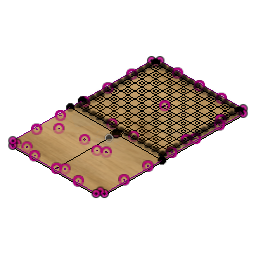
Bottom Plate (Autodesk Fusion 360 design; units mm, degrees)
Autodesk Fusion 360 part; units mm, degrees
note: some values were not read from the file. Set by a fixed rule: which sketch regions a step uses.
sketch "Sketch1" plane through (0, 0, 0) normal (0, 1, 0) x (1, 0, 0)
  line L0 (0, 0) -> (330, 0)
  line L1 (330, 0) -> (330, -530)
  line L2 (330, -530) -> (0, -530)
  line L3 (0, -530) -> (0, 0)
  dimension "d1" = 530
  dimension "d2" = 330
  measures "d1" distance of L0.start
extrude "Extrude1" add sketch "Sketch1" along normal blind 6
sketch "Sketch3" plane through (0, 6, 0) normal (0, 1, 0) x (-1, 0, 0)
  circle A0 centre (-7.5, 7.5) radius 1.5
  line L0 (0, 0) -> (0, 530)
  line L1 (-330, 0) -> (0, 0)
  circle A1 centre (-322.5, 7.5) radius 1.5
  circle A2 centre (-7.5, 93.3333) radius 1.5
  circle A3 centre (-322.5, 93.3333) radius 1.5
  circle A4 centre (-7.5, 179.1667) radius 1.5
  circle A5 centre (-322.5, 179.1667) radius 1.5
  circle A6 centre (-7.5, 265) radius 1.5
  circle A7 centre (-322.5, 265) radius 1.5
  circle A8 centre (-7.5, 350.8333) radius 1.5
  circle A9 centre (-322.5, 350.8333) radius 1.5
  circle A10 centre (-7.5, 436.6667) radius 1.5
  circle A11 centre (-322.5, 436.6667) radius 1.5
  circle A12 centre (-7.5, 522.5) radius 1.5
  circle A13 centre (-322.5, 522.5) radius 1.5
  circle A14 centre (-243.75, 7.5) radius 1.5
  circle A15 centre (-165, 7.5) radius 1.5
  circle A16 centre (-86.25, 7.5) radius 1.5
  circle A17 centre (-7.5, 7.5) radius 1.5
  circle A18 centre (-322.5, 522.5) radius 1.5
  circle A19 centre (-243.75, 522.5) radius 1.5
  circle A20 centre (-165, 522.5) radius 1.5
  circle A21 centre (-86.25, 522.5) radius 1.5
  circle A22 centre (-7.5, 522.5) radius 1.5
  dimension "d87" = 3
  dimension "d88" = 7.5
  dimension "d89" = 7.5
  dimension "d92" = -315
  dimension "d93" = 515
  dimension "d96" = 315
  dimension "d97" = 515
  measures "d87" diameter of A0
  measures "d88" distance of L0
extrude "Extrude3" cut sketch "Sketch3" against normal through all
sketch "Sketch4" plane through (0, 6, 0) normal (0, 1, 0) x (-1, 0, 0)
  line L0 (0, 530) -> (-330, 530)
  line L1 (-330, 530) -> (-330, 0)
  line L2 (-330, 0) -> (0, 0)
  line L3 (0, 0) -> (0, 530)
  line L4 (0, 530) -> (-15, 530)
  line L5 (-15, 530) -> (-15, 515)
  line L6 (-15, 515) -> (0, 515)
  line L7 (0, 515) -> (0, 530)
  line L8 (-330, 530) -> (-315, 530)
  line L9 (-315, 530) -> (-315, 515)
  line L10 (-315, 515) -> (-330, 515)
  line L11 (-330, 515) -> (-330, 530)
  line L12 (-330, 0) -> (-315, 0)
  line L13 (-315, 0) -> (-315, 15)
  line L14 (-315, 15) -> (-330, 15)
  line L15 (-330, 15) -> (-330, 0)
  line L16 (0, 0) -> (-15, 0)
  line L17 (-15, 0) -> (-15, 15)
  line L18 (-15, 15) -> (0, 15)
  line L19 (0, 15) -> (0, 0)
  circle A0 centre (-7.5, 265) radius 1.5
  circle A1 centre (-86.25, 7.5) radius 1.5
  circle A2 centre (-322.5, 93.3333) radius 1.5
  circle A3 centre (-322.5, 436.6667) radius 1.5
  circle A4 centre (-86.25, 522.5) radius 1.5
  circle A5 centre (-165, 522.5) radius 1.5
  circle A6 centre (-322.5, 350.8333) radius 1.5
  circle A7 centre (-322.5, 7.5) radius 1.5
  circle A8 centre (-7.5, 7.5) radius 1.5
  circle A9 centre (-7.5, 350.8333) radius 1.5
  circle A10 centre (-7.5, 179.1667) radius 1.5
  circle A11 centre (-165, 7.5) radius 1.5
  circle A12 centre (-322.5, 179.1667) radius 1.5
  circle A13 centre (-322.5, 522.5) radius 1.5
  circle A14 centre (-7.5, 522.5) radius 1.5
  circle A15 centre (-243.75, 522.5) radius 1.5
  circle A16 centre (-322.5, 265) radius 1.5
  circle A17 centre (-243.75, 7.5) radius 1.5
  circle A18 centre (-7.5, 93.3333) radius 1.5
  circle A19 centre (-7.5, 436.6667) radius 1.5
  dimension "d38" = 15
  dimension "d39" = 15
  dimension "d40" = 15
  dimension "d41" = 15
  dimension "d42" = 15
  dimension "d43" = 15
  dimension "d44" = 15
  dimension "d45" = 15
  measures "d44" distance of L2.end
  measures "d45" distance of L2.end
extrude "Extrude4" cut sketch "Sketch4" against normal blind 25 contours L0 L3 L4 L5 L6 L7 | L0 L1 L8 L9 L10 L11 | L2 L3 L16 L17 L18 L19 | L1 L2 L12 L13 L14 L15
sketch "Sketch5" plane through (0, 6, 0) normal (0, 1, 0) x (-1, 0, 0)
  line L0 (-315, 530) -> (-315, 515)
  line L1 (-315, 515) -> (-330, 515)
  line L2 (-330, 515) -> (-330, 15)
  line L3 (-330, 15) -> (-315, 15)
  line L4 (-315, 15) -> (-315, 0)
  line L5 (-315, 0) -> (-15, 0)
  line L6 (-15, 0) -> (-15, 15)
  line L7 (-15, 15) -> (0, 15)
  line L8 (0, 15) -> (0, 515)
  line L9 (0, 515) -> (-15, 515)
  line L10 (-15, 515) -> (-15, 530)
  line L11 (-15, 530) -> (-315, 530)
  line L12 (-126, 382) -> (-204, 382)
  line L13 (-204, 382) -> (-204, 284)
  line L14 (-204, 284) -> (-126, 284)
  line L15 (-126, 284) -> (-126, 382)
  circle A0 centre (-126, 382) radius 2.5
  circle A1 centre (-126, 284) radius 2.5
  circle A2 centre (-204, 284) radius 2.5
  circle A3 centre (-204, 382) radius 2.5
  line L16 (-165, 530) -> (-165, 382) construction
  circle A4 centre (-7.5, 436.6667) radius 1.5
  circle A5 centre (-7.5, 93.3333) radius 1.5
  circle A6 centre (-243.75, 7.5) radius 1.5
  circle A7 centre (-322.5, 265) radius 1.5
  circle A8 centre (-243.75, 522.5) radius 1.5
  circle A9 centre (-322.5, 179.1667) radius 1.5
  circle A10 centre (-165, 7.5) radius 1.5
  circle A11 centre (-7.5, 179.1667) radius 1.5
  circle A12 centre (-7.5, 350.8333) radius 1.5
  circle A13 centre (-322.5, 350.8333) radius 1.5
  circle A14 centre (-165, 522.5) radius 1.5
  circle A15 centre (-86.25, 522.5) radius 1.5
  circle A16 centre (-322.5, 436.6667) radius 1.5
  circle A17 centre (-322.5, 93.3333) radius 1.5
  circle A18 centre (-86.25, 7.5) radius 1.5
  circle A19 centre (-7.5, 265) radius 1.5
  dimension "d48" = 78
  dimension "d49" = 98
  dimension "d50" = 5
  dimension "d51" = 5
  dimension "d52" = 5
  dimension "d53" = 5
  dimension "d54" = 148
  measures "d49" distance of origin
  measures "d50" diameter of A0
  measures "d51" diameter of A1
  measures "d52" diameter of A2
  measures "d53" diameter of A3
extrude "Extrude5" cut sketch "Sketch5" against normal through all contours L12 L13 A3 | L12 L13 A3 | L12 L15 A0 | L12 L15 A0 | L13 L14 A2 | L13 L14 A2 | L14 L15 A1 | L14 L15 A1
sketch "Sketch6" plane through (0, 6, 0) normal (0, 1, 0) x (-1, 0, 0)
  circle A0 centre (-204, 284) radius 2.5
  circle A1 centre (-204, 382) radius 2.5
  circle A2 centre (-126, 284) radius 2.5
  circle A3 centre (-126, 382) radius 2.5
  line L0 (-315, 530) -> (-315, 515)
  line L1 (-315, 515) -> (-330, 515)
  line L2 (-330, 515) -> (-330, 15)
  line L3 (-330, 15) -> (-315, 15)
  line L4 (-315, 15) -> (-315, 0)
  line L5 (-315, 0) -> (-15, 0)
  line L6 (-15, 0) -> (-15, 15)
  line L7 (-15, 15) -> (0, 15)
  line L8 (0, 15) -> (0, 515)
  line L9 (0, 515) -> (-15, 515)
  line L10 (-15, 515) -> (-15, 530)
  line L11 (-15, 530) -> (-315, 530)
  line L12 (-45, 509) -> (-182, 509) construction
  line L13 (-182, 509) -> (-182, 394) construction
  line L14 (-182, 394) -> (-45, 394) construction
  line L15 (-45, 394) -> (-45, 509) construction
  circle A4 centre (-182, 509) radius 2
  circle A5 centre (-45, 509) radius 2
  circle A6 centre (-45, 394) radius 2
  circle A7 centre (-182, 394) radius 2
  circle A8 centre (-7.5, 436.6667) radius 1.5
  circle A9 centre (-7.5, 93.3333) radius 1.5
  circle A10 centre (-243.75, 7.5) radius 1.5
  circle A11 centre (-322.5, 265) radius 1.5
  circle A12 centre (-243.75, 522.5) radius 1.5
  circle A13 centre (-322.5, 179.1667) radius 1.5
  circle A14 centre (-165, 7.5) radius 1.5
  circle A15 centre (-7.5, 179.1667) radius 1.5
  circle A16 centre (-7.5, 350.8333) radius 1.5
  circle A17 centre (-322.5, 350.8333) radius 1.5
  circle A18 centre (-165, 522.5) radius 1.5
  circle A19 centre (-86.25, 522.5) radius 1.5
  circle A20 centre (-322.5, 436.6667) radius 1.5
  circle A21 centre (-322.5, 93.3333) radius 1.5
  circle A22 centre (-86.25, 7.5) radius 1.5
  circle A23 centre (-7.5, 265) radius 1.5
  dimension "d56" = 115
  dimension "d57" = 137
  dimension "d58" = 4
  dimension "d59" = 21
  dimension "d60" = 45
  measures "d58" diameter of A4
  measures "d59" distance of L11 L12
  measures "d60" distance of L8 L15
extrude "Extrude6" cut sketch "Sketch6" against normal through all contours A4 | A5 | A6 | A7
sketch "Sketch9" plane through (0, 6, 0) normal (0, 1, 0) x (-1, 0, 0)
  circle A0 centre (-45, 394) radius 2
  circle A1 centre (-182, 394) radius 2
  circle A2 centre (-45, 509) radius 2
  circle A3 centre (-182, 509) radius 2
  circle A4 centre (-204, 284) radius 2.5
  circle A5 centre (-204, 382) radius 2.5
  circle A6 centre (-126, 284) radius 2.5
  circle A7 centre (-126, 382) radius 2.5
  circle A8 centre (-7.5, 436.6667) radius 1.5
  circle A9 centre (-7.5, 93.3333) radius 1.5
  circle A10 centre (-243.75, 7.5) radius 1.5
  circle A11 centre (-322.5, 265) radius 1.5
  circle A12 centre (-243.75, 522.5) radius 1.5
  circle A13 centre (-322.5, 179.1667) radius 1.5
  circle A14 centre (-165, 7.5) radius 1.5
  circle A15 centre (-7.5, 179.1667) radius 1.5
  circle A16 centre (-7.5, 350.8333) radius 1.5
  circle A17 centre (-322.5, 350.8333) radius 1.5
  circle A18 centre (-165, 522.5) radius 1.5
  circle A19 centre (-86.25, 522.5) radius 1.5
  circle A20 centre (-322.5, 436.6667) radius 1.5
  circle A21 centre (-322.5, 93.3333) radius 1.5
  circle A22 centre (-86.25, 7.5) radius 1.5
  circle A23 centre (-7.5, 265) radius 1.5
  line L0 (-315, 530) -> (-315, 515)
  line L1 (-315, 515) -> (-330, 515)
  line L2 (-330, 515) -> (-330, 15)
  line L3 (-330, 15) -> (-315, 15)
  line L4 (-315, 15) -> (-315, 0)
  line L5 (-315, 0) -> (-15, 0)
  line L6 (-15, 0) -> (-15, 15)
  line L7 (-15, 15) -> (0, 15)
  line L8 (0, 15) -> (0, 515)
  line L9 (0, 515) -> (-15, 515)
  line L10 (-15, 515) -> (-15, 530)
  line L11 (-15, 530) -> (-315, 530)
  circle A24 centre (-310, 75) radius 2
  circle A25 centre (-310, 200) radius 2
  circle A26 centre (-165, 132.643) radius 2.5
  line L12 (-126, 284) -> (-126, 382) construction
  line L13 (-204, 284) -> (-204, 382) construction
  line L14 (-204, 333) -> (-126, 333) construction
  line L15 (-165, 307.643) -> (-165, 132.643) construction
  line L16 (-165, 307.643) -> (-165, 333) construction
  circle A27 centre (-165, 307.643) radius 15 construction
  dimension "d98" = 4
  dimension "d99" = 4
  dimension "d100" = 20
  dimension "d101" = 20
  dimension "d102" = 75
  dimension "d103" = 200
  dimension "d104" = 5
  dimension "d105" = 175
  dimension "d108" = 23.643
  dimension "d109" = 30
  measures "d98" diameter of A24
  measures "d99" diameter of A25
  measures "d104" diameter of A26
  measures "d109" diameter of A27
extrude "Extrude7" cut sketch "Sketch9" against normal blind 10 contours A24 | A25 | A26
sketch "Sketch7" plane through (0, 6, 0) normal (0, 1, 0) x (-1, 0, 0)
  circle A0 centre (-45, 394) radius 2
  circle A1 centre (-182, 394) radius 2
  circle A2 centre (-45, 509) radius 2
  circle A3 centre (-182, 509) radius 2
  circle A4 centre (-204, 284) radius 2.5
  circle A5 centre (-204, 382) radius 2.5
  circle A6 centre (-126, 284) radius 2.5
  circle A7 centre (-126, 382) radius 2.5
  line L0 (-315, 530) -> (-315, 515)
  line L1 (-315, 515) -> (-330, 515)
  line L2 (-330, 515) -> (-330, 15)
  line L3 (-330, 15) -> (-315, 15)
  line L4 (-315, 15) -> (-315, 0)
  line L5 (-315, 0) -> (-15, 0)
  line L6 (-15, 0) -> (-15, 15)
  line L7 (-15, 15) -> (0, 15)
  line L8 (0, 15) -> (0, 515)
  line L9 (0, 515) -> (-15, 515)
  line L10 (-15, 515) -> (-15, 530)
  line L11 (-15, 530) -> (-315, 530)
  line L12 (-15, 15) -> (-315, 15)
  line L13 (-315, 15) -> (-315, 290)
  line L14 (-315, 290) -> (-15, 290)
  line L15 (-15, 290) -> (-15, 15)
  line L16 (-15, 40) -> (-315, 40)
  line L17 (-15, 65) -> (-315, 65)
  line L18 (-15, 90) -> (-315, 90)
  line L19 (-15, 115) -> (-315, 115)
  line L20 (-15, 140) -> (-315, 140)
  line L21 (-15, 165) -> (-315, 165)
  line L22 (-15, 190) -> (-315, 190)
  line L23 (-15, 215) -> (-315, 215)
  line L24 (-15, 240) -> (-315, 240)
  line L25 (-15, 265) -> (-315, 265)
  line L26 (-32.5, 32.5) -> (-22.5, 32.5)
  line L27 (-22.5, 32.5) -> (-22.5, 22.5)
  line L28 (-22.5, 22.5) -> (-32.5, 22.5)
  line L29 (-32.5, 22.5) -> (-32.5, 32.5)
  line L30 (-15, 290) -> (-315, 290)
  line L31 (-40, 290) -> (-40, 15)
  line L32 (-65, 290) -> (-65, 15)
  line L33 (-90, 290) -> (-90, 15)
  line L34 (-115, 290) -> (-115, 15)
  line L35 (-140, 290) -> (-140, 15)
  line L36 (-165, 290) -> (-165, 15)
  line L37 (-190, 290) -> (-190, 15)
  line L38 (-215, 290) -> (-215, 15)
  line L39 (-240, 290) -> (-240, 15)
  line L40 (-265, 290) -> (-265, 15)
  line L41 (-290, 290) -> (-290, 15)
  line L42 (-315, 290) -> (-315, 15)
  line L43 (-72.5, 22.5) -> (-82.5, 22.5)
  line L44 (-72.5, 32.5) -> (-72.5, 22.5)
  line L45 (-82.5, 32.5) -> (-72.5, 32.5)
  line L46 (-82.5, 22.5) -> (-82.5, 32.5)
  line L47 (-122.5, 22.5) -> (-132.5, 22.5)
  line L48 (-122.5, 32.5) -> (-122.5, 22.5)
  line L49 (-132.5, 32.5) -> (-122.5, 32.5)
  line L50 (-132.5, 22.5) -> (-132.5, 32.5)
  line L51 (-172.5, 22.5) -> (-182.5, 22.5)
  line L52 (-172.5, 32.5) -> (-172.5, 22.5)
  line L53 (-182.5, 32.5) -> (-172.5, 32.5)
  line L54 (-182.5, 22.5) -> (-182.5, 32.5)
  line L55 (-222.5, 22.5) -> (-232.5, 22.5)
  line L56 (-222.5, 32.5) -> (-222.5, 22.5)
  line L57 (-232.5, 32.5) -> (-222.5, 32.5)
  line L58 (-232.5, 22.5) -> (-232.5, 32.5)
  line L59 (-272.5, 22.5) -> (-282.5, 22.5)
  line L60 (-272.5, 32.5) -> (-272.5, 22.5)
  line L61 (-282.5, 32.5) -> (-272.5, 32.5)
  line L62 (-282.5, 22.5) -> (-282.5, 32.5)
  line L63 (-22.5, 72.5) -> (-32.5, 72.5)
  line L64 (-22.5, 82.5) -> (-22.5, 72.5)
  line L65 (-32.5, 82.5) -> (-22.5, 82.5)
  line L66 (-32.5, 72.5) -> (-32.5, 82.5)
  line L67 (-72.5, 72.5) -> (-82.5, 72.5)
  line L68 (-72.5, 82.5) -> (-72.5, 72.5)
  line L69 (-82.5, 82.5) -> (-72.5, 82.5)
  line L70 (-82.5, 72.5) -> (-82.5, 82.5)
  line L71 (-122.5, 72.5) -> (-132.5, 72.5)
  line L72 (-122.5, 82.5) -> (-122.5, 72.5)
  line L73 (-132.5, 82.5) -> (-122.5, 82.5)
  line L74 (-132.5, 72.5) -> (-132.5, 82.5)
  line L75 (-172.5, 72.5) -> (-182.5, 72.5)
  line L76 (-172.5, 82.5) -> (-172.5, 72.5)
  line L77 (-182.5, 82.5) -> (-172.5, 82.5)
  line L78 (-182.5, 72.5) -> (-182.5, 82.5)
  line L79 (-222.5, 72.5) -> (-232.5, 72.5)
  line L80 (-222.5, 82.5) -> (-222.5, 72.5)
  line L81 (-232.5, 82.5) -> (-222.5, 82.5)
  line L82 (-232.5, 72.5) -> (-232.5, 82.5)
  line L83 (-272.5, 72.5) -> (-282.5, 72.5)
  line L84 (-272.5, 82.5) -> (-272.5, 72.5)
  line L85 (-282.5, 82.5) -> (-272.5, 82.5)
  line L86 (-282.5, 72.5) -> (-282.5, 82.5)
  line L87 (-22.5, 122.5) -> (-32.5, 122.5)
  line L88 (-22.5, 132.5) -> (-22.5, 122.5)
  line L89 (-32.5, 132.5) -> (-22.5, 132.5)
  line L90 (-32.5, 122.5) -> (-32.5, 132.5)
  line L91 (-72.5, 122.5) -> (-82.5, 122.5)
  line L92 (-72.5, 132.5) -> (-72.5, 122.5)
  line L93 (-82.5, 132.5) -> (-72.5, 132.5)
  line L94 (-82.5, 122.5) -> (-82.5, 132.5)
  line L95 (-122.5, 122.5) -> (-132.5, 122.5)
  line L96 (-122.5, 132.5) -> (-122.5, 122.5)
  line L97 (-132.5, 132.5) -> (-122.5, 132.5)
  line L98 (-132.5, 122.5) -> (-132.5, 132.5)
  line L99 (-172.5, 122.5) -> (-182.5, 122.5)
  line L100 (-172.5, 132.5) -> (-172.5, 122.5)
  line L101 (-182.5, 132.5) -> (-172.5, 132.5)
  line L102 (-182.5, 122.5) -> (-182.5, 132.5)
  line L103 (-222.5, 122.5) -> (-232.5, 122.5)
  line L104 (-222.5, 132.5) -> (-222.5, 122.5)
  line L105 (-232.5, 132.5) -> (-222.5, 132.5)
  line L106 (-232.5, 122.5) -> (-232.5, 132.5)
  line L107 (-272.5, 122.5) -> (-282.5, 122.5)
  line L108 (-272.5, 132.5) -> (-272.5, 122.5)
  line L109 (-282.5, 132.5) -> (-272.5, 132.5)
  line L110 (-282.5, 122.5) -> (-282.5, 132.5)
  line L111 (-22.5, 172.5) -> (-32.5, 172.5)
  line L112 (-22.5, 182.5) -> (-22.5, 172.5)
  line L113 (-32.5, 182.5) -> (-22.5, 182.5)
  line L114 (-32.5, 172.5) -> (-32.5, 182.5)
  line L115 (-72.5, 172.5) -> (-82.5, 172.5)
  line L116 (-72.5, 182.5) -> (-72.5, 172.5)
  line L117 (-82.5, 182.5) -> (-72.5, 182.5)
  line L118 (-82.5, 172.5) -> (-82.5, 182.5)
  line L119 (-122.5, 172.5) -> (-132.5, 172.5)
  line L120 (-122.5, 182.5) -> (-122.5, 172.5)
  line L121 (-132.5, 182.5) -> (-122.5, 182.5)
  line L122 (-132.5, 172.5) -> (-132.5, 182.5)
  line L123 (-172.5, 172.5) -> (-182.5, 172.5)
  line L124 (-172.5, 182.5) -> (-172.5, 172.5)
  line L125 (-182.5, 182.5) -> (-172.5, 182.5)
  line L126 (-182.5, 172.5) -> (-182.5, 182.5)
  line L127 (-222.5, 172.5) -> (-232.5, 172.5)
  line L128 (-222.5, 182.5) -> (-222.5, 172.5)
  line L129 (-232.5, 182.5) -> (-222.5, 182.5)
  line L130 (-232.5, 172.5) -> (-232.5, 182.5)
  line L131 (-272.5, 172.5) -> (-282.5, 172.5)
  line L132 (-272.5, 182.5) -> (-272.5, 172.5)
  line L133 (-282.5, 182.5) -> (-272.5, 182.5)
  line L134 (-282.5, 172.5) -> (-282.5, 182.5)
  line L135 (-22.5, 222.5) -> (-32.5, 222.5)
  line L136 (-22.5, 232.5) -> (-22.5, 222.5)
  line L137 (-32.5, 232.5) -> (-22.5, 232.5)
  line L138 (-32.5, 222.5) -> (-32.5, 232.5)
  line L139 (-72.5, 222.5) -> (-82.5, 222.5)
  line L140 (-72.5, 232.5) -> (-72.5, 222.5)
  line L141 (-82.5, 232.5) -> (-72.5, 232.5)
  line L142 (-82.5, 222.5) -> (-82.5, 232.5)
  line L143 (-122.5, 222.5) -> (-132.5, 222.5)
  line L144 (-122.5, 232.5) -> (-122.5, 222.5)
  line L145 (-132.5, 232.5) -> (-122.5, 232.5)
  line L146 (-132.5, 222.5) -> (-132.5, 232.5)
  line L147 (-172.5, 222.5) -> (-182.5, 222.5)
  line L148 (-172.5, 232.5) -> (-172.5, 222.5)
  line L149 (-182.5, 232.5) -> (-172.5, 232.5)
  line L150 (-182.5, 222.5) -> (-182.5, 232.5)
  line L151 (-222.5, 222.5) -> (-232.5, 222.5)
  line L152 (-222.5, 232.5) -> (-222.5, 222.5)
  line L153 (-232.5, 232.5) -> (-222.5, 232.5)
  line L154 (-232.5, 222.5) -> (-232.5, 232.5)
  line L155 (-272.5, 222.5) -> (-282.5, 222.5)
  line L156 (-272.5, 232.5) -> (-272.5, 222.5)
  line L157 (-282.5, 232.5) -> (-272.5, 232.5)
  line L158 (-282.5, 222.5) -> (-282.5, 232.5)
  line L159 (-22.5, 272.5) -> (-32.5, 272.5)
  line L160 (-22.5, 282.5) -> (-22.5, 272.5)
  line L161 (-32.5, 282.5) -> (-22.5, 282.5)
  line L162 (-32.5, 272.5) -> (-32.5, 282.5)
  line L163 (-72.5, 272.5) -> (-82.5, 272.5)
  line L164 (-72.5, 282.5) -> (-72.5, 272.5)
  line L165 (-82.5, 282.5) -> (-72.5, 282.5)
  line L166 (-82.5, 272.5) -> (-82.5, 282.5)
  line L167 (-122.5, 272.5) -> (-132.5, 272.5)
  line L168 (-122.5, 282.5) -> (-122.5, 272.5)
  line L169 (-132.5, 282.5) -> (-122.5, 282.5)
  line L170 (-132.5, 272.5) -> (-132.5, 282.5)
  line L171 (-172.5, 272.5) -> (-182.5, 272.5)
  line L172 (-172.5, 282.5) -> (-172.5, 272.5)
  line L173 (-182.5, 282.5) -> (-172.5, 282.5)
  line L174 (-182.5, 272.5) -> (-182.5, 282.5)
  line L175 (-222.5, 272.5) -> (-232.5, 272.5)
  line L176 (-222.5, 282.5) -> (-222.5, 272.5)
  line L177 (-232.5, 282.5) -> (-222.5, 282.5)
  line L178 (-232.5, 272.5) -> (-232.5, 282.5)
  line L179 (-272.5, 272.5) -> (-282.5, 272.5)
  line L180 (-272.5, 282.5) -> (-272.5, 272.5)
  line L181 (-282.5, 282.5) -> (-272.5, 282.5)
  line L182 (-282.5, 272.5) -> (-282.5, 282.5)
  line L183 (-47.5, 47.5) -> (-57.5, 47.5)
  line L184 (-57.5, 47.5) -> (-57.5, 57.5)
  line L185 (-57.5, 57.5) -> (-47.5, 57.5)
  line L186 (-47.5, 57.5) -> (-47.5, 47.5)
  line L187 (-107.5, 47.5) -> (-107.5, 57.5)
  line L188 (-97.5, 47.5) -> (-107.5, 47.5)
  line L189 (-97.5, 57.5) -> (-97.5, 47.5)
  line L190 (-107.5, 57.5) -> (-97.5, 57.5)
  line L191 (-157.5, 47.5) -> (-157.5, 57.5)
  line L192 (-147.5, 47.5) -> (-157.5, 47.5)
  line L193 (-147.5, 57.5) -> (-147.5, 47.5)
  line L194 (-157.5, 57.5) -> (-147.5, 57.5)
  line L195 (-207.5, 47.5) -> (-207.5, 57.5)
  line L196 (-197.5, 47.5) -> (-207.5, 47.5)
  line L197 (-197.5, 57.5) -> (-197.5, 47.5)
  line L198 (-207.5, 57.5) -> (-197.5, 57.5)
  line L199 (-57.5, 97.5) -> (-57.5, 107.5)
  line L200 (-47.5, 97.5) -> (-57.5, 97.5)
  line L201 (-47.5, 107.5) -> (-47.5, 97.5)
  line L202 (-57.5, 107.5) -> (-47.5, 107.5)
  line L203 (-107.5, 97.5) -> (-107.5, 107.5)
  line L204 (-97.5, 97.5) -> (-107.5, 97.5)
  line L205 (-97.5, 107.5) -> (-97.5, 97.5)
  line L206 (-107.5, 107.5) -> (-97.5, 107.5)
  line L207 (-157.5, 97.5) -> (-157.5, 107.5)
  line L208 (-147.5, 97.5) -> (-157.5, 97.5)
  line L209 (-147.5, 107.5) -> (-147.5, 97.5)
  line L210 (-157.5, 107.5) -> (-147.5, 107.5)
  line L211 (-207.5, 97.5) -> (-207.5, 107.5)
  line L212 (-197.5, 97.5) -> (-207.5, 97.5)
  line L213 (-197.5, 107.5) -> (-197.5, 97.5)
  line L214 (-207.5, 107.5) -> (-197.5, 107.5)
  line L215 (-57.5, 147.5) -> (-57.5, 157.5)
  line L216 (-47.5, 147.5) -> (-57.5, 147.5)
  line L217 (-47.5, 157.5) -> (-47.5, 147.5)
  line L218 (-57.5, 157.5) -> (-47.5, 157.5)
  line L219 (-107.5, 147.5) -> (-107.5, 157.5)
  line L220 (-97.5, 147.5) -> (-107.5, 147.5)
  line L221 (-97.5, 157.5) -> (-97.5, 147.5)
  line L222 (-107.5, 157.5) -> (-97.5, 157.5)
  line L223 (-157.5, 147.5) -> (-157.5, 157.5)
  line L224 (-147.5, 147.5) -> (-157.5, 147.5)
  line L225 (-147.5, 157.5) -> (-147.5, 147.5)
  line L226 (-157.5, 157.5) -> (-147.5, 157.5)
  line L227 (-207.5, 147.5) -> (-207.5, 157.5)
  line L228 (-197.5, 147.5) -> (-207.5, 147.5)
  line L229 (-197.5, 157.5) -> (-197.5, 147.5)
  line L230 (-207.5, 157.5) -> (-197.5, 157.5)
  line L231 (-57.5, 197.5) -> (-57.5, 207.5)
  line L232 (-47.5, 197.5) -> (-57.5, 197.5)
  line L233 (-47.5, 207.5) -> (-47.5, 197.5)
  line L234 (-57.5, 207.5) -> (-47.5, 207.5)
  line L235 (-107.5, 197.5) -> (-107.5, 207.5)
  line L236 (-97.5, 197.5) -> (-107.5, 197.5)
  line L237 (-97.5, 207.5) -> (-97.5, 197.5)
  line L238 (-107.5, 207.5) -> (-97.5, 207.5)
  line L239 (-157.5, 197.5) -> (-157.5, 207.5)
  line L240 (-147.5, 197.5) -> (-157.5, 197.5)
  line L241 (-147.5, 207.5) -> (-147.5, 197.5)
  line L242 (-157.5, 207.5) -> (-147.5, 207.5)
  line L243 (-207.5, 197.5) -> (-207.5, 207.5)
  line L244 (-197.5, 197.5) -> (-207.5, 197.5)
  line L245 (-197.5, 207.5) -> (-197.5, 197.5)
  line L246 (-207.5, 207.5) -> (-197.5, 207.5)
  line L247 (-57.5, 247.5) -> (-57.5, 257.5)
  line L248 (-47.5, 247.5) -> (-57.5, 247.5)
  line L249 (-47.5, 257.5) -> (-47.5, 247.5)
  line L250 (-57.5, 257.5) -> (-47.5, 257.5)
  line L251 (-107.5, 247.5) -> (-107.5, 257.5)
  line L252 (-97.5, 247.5) -> (-107.5, 247.5)
  line L253 (-97.5, 257.5) -> (-97.5, 247.5)
  line L254 (-107.5, 257.5) -> (-97.5, 257.5)
  line L255 (-157.5, 247.5) -> (-157.5, 257.5)
  line L256 (-147.5, 247.5) -> (-157.5, 247.5)
  line L257 (-147.5, 257.5) -> (-147.5, 247.5)
  line L258 (-157.5, 257.5) -> (-147.5, 257.5)
  line L259 (-207.5, 247.5) -> (-207.5, 257.5)
  line L260 (-197.5, 247.5) -> (-207.5, 247.5)
  line L261 (-197.5, 257.5) -> (-197.5, 247.5)
  line L262 (-207.5, 257.5) -> (-197.5, 257.5)
  line L263 (-257.5, 47.5) -> (-257.5, 57.5)
  line L264 (-247.5, 47.5) -> (-257.5, 47.5)
  line L265 (-247.5, 57.5) -> (-247.5, 47.5)
  line L266 (-257.5, 57.5) -> (-247.5, 57.5)
  line L267 (-307.5, 47.5) -> (-307.5, 57.5)
  line L268 (-297.5, 47.5) -> (-307.5, 47.5)
  line L269 (-297.5, 57.5) -> (-297.5, 47.5)
  line L270 (-307.5, 57.5) -> (-297.5, 57.5)
  line L271 (-257.5, 97.5) -> (-257.5, 107.5)
  line L272 (-247.5, 97.5) -> (-257.5, 97.5)
  line L273 (-247.5, 107.5) -> (-247.5, 97.5)
  line L274 (-257.5, 107.5) -> (-247.5, 107.5)
  line L275 (-307.5, 97.5) -> (-307.5, 107.5)
  line L276 (-297.5, 97.5) -> (-307.5, 97.5)
  line L277 (-297.5, 107.5) -> (-297.5, 97.5)
  line L278 (-307.5, 107.5) -> (-297.5, 107.5)
  line L279 (-257.5, 147.5) -> (-257.5, 157.5)
  line L280 (-247.5, 147.5) -> (-257.5, 147.5)
  line L281 (-247.5, 157.5) -> (-247.5, 147.5)
  line L282 (-257.5, 157.5) -> (-247.5, 157.5)
  line L283 (-307.5, 147.5) -> (-307.5, 157.5)
  line L284 (-297.5, 147.5) -> (-307.5, 147.5)
  line L285 (-297.5, 157.5) -> (-297.5, 147.5)
  line L286 (-307.5, 157.5) -> (-297.5, 157.5)
  line L287 (-257.5, 197.5) -> (-257.5, 207.5)
  line L288 (-247.5, 197.5) -> (-257.5, 197.5)
  line L289 (-247.5, 207.5) -> (-247.5, 197.5)
  line L290 (-257.5, 207.5) -> (-247.5, 207.5)
  line L291 (-307.5, 197.5) -> (-307.5, 207.5)
  line L292 (-297.5, 197.5) -> (-307.5, 197.5)
  line L293 (-297.5, 207.5) -> (-297.5, 197.5)
  line L294 (-307.5, 207.5) -> (-297.5, 207.5)
  line L295 (-257.5, 247.5) -> (-257.5, 257.5)
  line L296 (-247.5, 247.5) -> (-257.5, 247.5)
  line L297 (-247.5, 257.5) -> (-247.5, 247.5)
  line L298 (-257.5, 257.5) -> (-247.5, 257.5)
  line L299 (-307.5, 247.5) -> (-307.5, 257.5)
  line L300 (-297.5, 247.5) -> (-307.5, 247.5)
  line L301 (-297.5, 257.5) -> (-297.5, 247.5)
  line L302 (-307.5, 257.5) -> (-297.5, 257.5)
  circle A8 centre (-7.5, 436.6667) radius 1.5
  circle A9 centre (-7.5, 93.3333) radius 1.5
  circle A10 centre (-243.75, 7.5) radius 1.5
  circle A11 centre (-322.5, 265) radius 1.5
  circle A12 centre (-243.75, 522.5) radius 1.5
  circle A13 centre (-322.5, 179.1667) radius 1.5
  circle A14 centre (-165, 7.5) radius 1.5
  circle A15 centre (-7.5, 179.1667) radius 1.5
  circle A16 centre (-7.5, 350.8333) radius 1.5
  circle A17 centre (-322.5, 350.8333) radius 1.5
  circle A18 centre (-165, 522.5) radius 1.5
  circle A19 centre (-86.25, 522.5) radius 1.5
  circle A20 centre (-322.5, 436.6667) radius 1.5
  circle A21 centre (-322.5, 93.3333) radius 1.5
  circle A22 centre (-86.25, 7.5) radius 1.5
  circle A23 centre (-7.5, 265) radius 1.5
  circle A24 centre (-45, 394) radius 2
  circle A25 centre (-182, 394) radius 2
  circle A26 centre (-45, 509) radius 2
  circle A27 centre (-182, 509) radius 2
  circle A28 centre (-204, 284) radius 2.5
  circle A29 centre (-204, 382) radius 2.5
  circle A30 centre (-126, 284) radius 2.5
  circle A31 centre (-126, 382) radius 2.5
  line L303 (-330, 515) -> (-315, 515)
  line L304 (-315, 515) -> (-315, 530)
  line L305 (-315, 530) -> (-15, 530)
  line L306 (-15, 530) -> (-15, 515)
  line L307 (-15, 515) -> (0, 515)
  line L308 (0, 515) -> (0, 15)
  line L309 (0, 15) -> (-15, 15)
  line L310 (-15, 15) -> (-15, 0)
  line L311 (-15, 0) -> (-315, 0)
  line L312 (-315, 0) -> (-315, 15)
  line L313 (-315, 15) -> (-330, 15)
  line L314 (-330, 15) -> (-330, 515)
  circle A32 centre (-7.5, 436.6667) radius 1.5
  circle A33 centre (-7.5, 93.3333) radius 1.5
  circle A34 centre (-243.75, 7.5) radius 1.5
  circle A35 centre (-322.5, 265) radius 1.5
  circle A36 centre (-243.75, 522.5) radius 1.5
  circle A37 centre (-322.5, 179.1667) radius 1.5
  circle A38 centre (-165, 7.5) radius 1.5
  circle A39 centre (-7.5, 179.1667) radius 1.5
  circle A40 centre (-7.5, 350.8333) radius 1.5
  circle A41 centre (-322.5, 350.8333) radius 1.5
  circle A42 centre (-165, 522.5) radius 1.5
  circle A43 centre (-86.25, 522.5) radius 1.5
  circle A44 centre (-322.5, 436.6667) radius 1.5
  circle A45 centre (-322.5, 93.3333) radius 1.5
  circle A46 centre (-86.25, 7.5) radius 1.5
  circle A47 centre (-7.5, 265) radius 1.5
  circle A48 centre (-165, 132.643) radius 2.5
  circle A49 centre (-310, 200) radius 2
  circle A50 centre (-310, 75) radius 2
  circle A51 centre (-165, 132.643) radius 2.5
  circle A52 centre (-310, 200) radius 2
  circle A53 centre (-310, 75) radius 2
  line L315 (-165, 307.643) -> (-165, 530)
  circle A54 centre (-165, 307.643) radius 15
  line L316 (0, 307.643) -> (-330, 307.643)
  point P0 (0, 28672)
  point P1 (0, 0)
  point P2 (0, 0)
  dimension "d62" = 275
  dimension "d65" = 0
  dimension "d66" = 275
  dimension "d69" = -300
  dimension "d70" = 0
  dimension "d71" = 10
  dimension "d72" = 10
  dimension "d73" = 7.5
  dimension "d74" = 7.5
  dimension "d77" = -250
  dimension "d78" = 250
  dimension "d79" = 10
  dimension "d80" = 10
  dimension "d81" = 7.5
  dimension "d82" = 7.5
  dimension "d85" = -250
  dimension "d86" = 200
  dimension "d110" = 30
  measures "d73" distance of L16 L26
  measures "d74" distance of L15 L27
  measures "d81" distance of L16 L183
  measures "d82" distance of L32 L184
  measures "d110" diameter of A54
equation "d54 = 15 mm + 133 mm"
equation "d59 = 15 mm + 6 mm"
equation "d60 = 30 mm + 15 mm"
